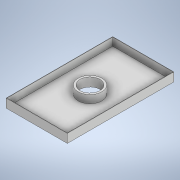
# Autodesk Inventor part: ЗЕМЛЯЕМКОСТЬ
Saved by Autodesk Inventor 2022.4 (Build 264492010, 492A)
## iProperties
Created: 2023-02-20
Part Number: ЗЕМЛЯЕМКОСТЬ
Material: Типовые
Document SubType Name: Modeling
Designer: artyo
Density: 1 g/cm^3
Appearance: По умолчанию
Author: artyo
Autodesk Inventor part; units mm, degrees
ref_plane "YZ Plane" through (0, 0, 0) normal (1, 0, 0) x (0, 1, 0)
ref_plane "XZ Plane" through (0, 0, 0) normal (0, 1, 0) x (-1, 0, 0)
ref_plane "XY Plane" through (0, 0, 0) normal (0, 0, 1) x (1, 0, 0)
sketch "Эскиз1" plane through (0, 0, 0) normal (0, 1, 0) x (-1, 0, 0)
  line L0 (-155, 270) -> (155, 270)
  line L1 (155, 270) -> (155, -270)
  line L2 (155, -270) -> (-155, -270)
  line L3 (-155, -270) -> (-155, 270)
  line L4 (-155, 270) -> (155, -270) construction
  line L5 (155, 270) -> (-155, -270) construction
  circle A0 centre (0, 0) radius 50
  dimension "d0" = 310
  dimension "d1" = 540
  dimension "d2" = 100
  constraints: 12 end point, 2 midpoint, 2 parallel, 1 centre point, 1 coincident, 1 horizontal, 1 perpendicular
  measures "d0" distance of L1.end L2.end
  measures "d1" distance of L0.end L1.end
  measures "d2" diameter of A0
extrude "Выдавливание1" add sketch "Эскиз1" along normal blind 4
sketch "Эскиз2" plane through (0, 4, 0) normal (0, 1, 0) x (1, 0, 0)
  line L0 (153, 268) -> (-153, 268)
  line L1 (-153, 268) -> (-153, -268)
  line L2 (-153, -268) -> (153, -268)
  line L3 (153, -268) -> (153, 268)
  line L4 (153, 268) -> (-153, -268) construction
  line L5 (-153, 268) -> (153, -268) construction
  line L6 (-155, 270) -> (-155, -270) projected
  line L7 (155, 270) -> (-155, 270)
  line L8 (-155, 270) -> (-155, -270)
  line L9 (-155, -270) -> (155, -270)
  line L10 (155, -270) -> (155, 270)
  line L11 (155, 270) -> (-155, -270) construction
  line L12 (-155, 270) -> (155, -270) construction
  point P0 (0, 0)
  dimension "d5" = 306
  dimension "d6" = 536
  constraints: 24 end point, 4 midpoint, 4 parallel, 2 horizontal, 2 perpendicular
  measures "d5" distance of L2.end L1.end
  measures "d6" distance of L1.end L0.end
extrude "Выдавливание2" add sketch "Эскиз2" along normal blind 40
sketch "Эскиз3" plane through (0, 4, 0) normal (0, 1, 0) x (1, 0, 0)
  circle A0 centre (0, 0) radius 50
  circle A1 centre (0, 0) radius 60
  dimension "d9" = 120
  constraints: 2 centre point, 2 coincident
  measures "d9" diameter of A1
extrude "Выдавливание3" add sketch "Эскиз3" along normal blind 40
